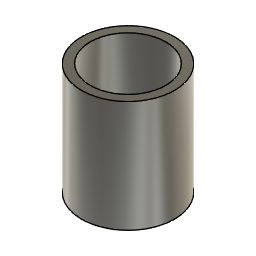
ExtensionCollar (Autodesk Fusion 360 design; units mm, degrees)
Autodesk Fusion 360 part; units mm, degrees
sketch "Sketch1" plane through (0, 0, 0) normal (0, 0, 1) x (1, 0, 0)
  circle A0 centre (0, 0) radius 25
  dimension "d5" = 50
  constraint coincident A0.centre origin
  measures "d5" diameter of A0
extrude "Extrude1" add sketch "Sketch1" along normal blind 10
sketch "Sketch2" plane through (0, 0, 10) normal (0, 0, 1) x (-1, 0, 0)
  circle A0 centre (0, 0) radius 25
  circle A1 centre (0, 0) radius 22.3
  dimension "d8" = 44.6
  constraint coincident A0.centre A1.centre
  measures "d8" diameter of A1
extrude "Extrude2" cut sketch "Sketch2" against normal blind 10 contours A1
sketch "Sketch3" plane through (0, 0, 10) normal (0, 0, 1) x (-1, 0, 0)
  circle A0 centre (0, 0) radius 22.3
  circle A1 centre (0, 0) radius 25
  circle A2 centre (0, 0) radius 25
  constraint coincident A0.centre A1.centre
extrude "Extrude3" add sketch "Sketch3" along normal blind 50 contours A0 | A1 A2
sketch "Sketch4" plane through (0, 0, 60) normal (0, 0, 1) x (-1, 0, 0)
  circle A0 centre (0, 0) radius 25
  circle A1 centre (0, 0) radius 20.3
  dimension "d13" = 40.6
  constraint coincident A0.centre A1.centre
  measures "d13" diameter of A1
extrude "Extrude4" cut sketch "Sketch4" against normal blind 50 contours A1
sketch "Sketch5" plane through (0, 0, 60) normal (0, 0, 1) x (-1, 0, 0)
  circle A0 centre (0, 0) radius 20.3
  circle A1 centre (0, 0) radius 25
  circle A2 centre (0, 0) radius 23.3
  dimension "d16" = 46.6
  constraint coincident A0.centre A1.centre
  measures "d16" diameter of A2
equation "LowerInnerDiam = 44 mm"
equation "Thickness = 3 mm"
equation "UpperInner = 40 mm"
equation "Tol = 0.6 mm"
equation "d5 = LowerInnerDiam + 2 * Thickness"
equation "d8 = LowerInnerDiam + Tol"
equation "d13 = 40 mm + Tol"
equation "d16 = UpperInner + Tol + 2 * Thickness"
